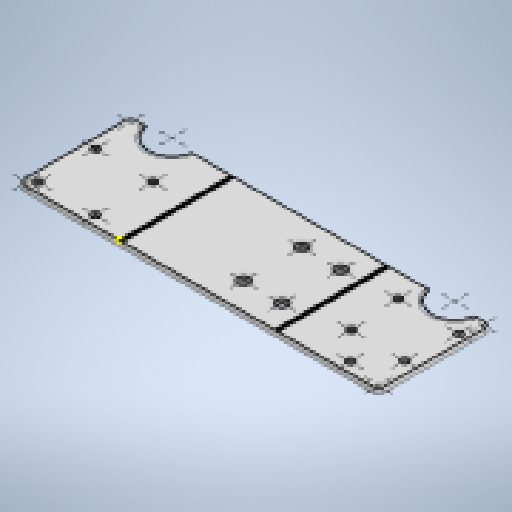
# Autodesk Inventor part: axis_22_bottom_frame
Saved by Autodesk Inventor 2026.1 (Build 301233000, 233)
## iProperties
Created: 2025-08-10
Part Number: axis_22_bottom_frame
Material: Generic
Document SubType Name: Modeling
Designer: LG
Density: 1 g/cm^3
Appearance: Default
Author: LG
Autodesk Inventor part; units mm, degrees
ref_plane "YZ Plane" through (0, 0, 0) normal (1, 0, 0) x (0, 1, 0)
ref_plane "XZ Plane" through (0, 0, 0) normal (0, 1, 0) x (-1, 0, 0)
ref_plane "XY Plane" through (0, 0, 0) normal (0, 0, 1) x (1, 0, 0)
sketch "Sketch1" plane through (0, 0, 0) normal (0, 1, 0) x (-1, 0, 0)
  line L0 (-0.4496, -29.3) -> (-0.4496, 0)
  line L1 (-41.2289, 0) -> (-41.2289, -29.3)
  circle A0 centre (-49.9386, -23.2) radius 1.05
  circle A1 centre (-50.9386, -9.98) radius 1.05
  circle A2 centre (-57.9386, -2.68) radius 1.05
  circle A3 centre (-64.9386, -9.98) radius 1.05
  circle A4 centre (-65.9386, -23.2) radius 1.05
  circle A5 centre (23.785, -2.5) radius 1.05
  circle A6 centre (8.735, -2.5) radius 1.05
  circle A7 centre (23.785, -17.6) radius 1.05
  circle A8 centre (8.735, -17.6) radius 1.05
  circle A9 centre (-25.6393, -7) radius 1.55
  circle A10 centre (-35.7793, -7) radius 1.55
  circle A11 centre (-25.6393, -22.3) radius 1.55
  circle A12 centre (-35.7793, -22.3) radius 1.55
  arc A13 (-67.0086, 0) -> (-68.0086, -1) centre (-67.0086, -1) ccw
  line L2 (-67.0086, 0) -> (25.33, 0)
  line L3 (-68.0086, -28.3) -> (-68.0086, -1)
  arc A14 (-68.0086, -28.3) -> (-67.0086, -29.3) centre (-67.0086, -28.3) ccw
  line L4 (-63.885, -29.3) -> (-67.0086, -29.3)
  arc A15 (-51.9921, -29.3) -> (-63.885, -29.3) centre (-57.9386, -30.1) ccw
  line L5 (10.3136, -29.3) -> (-51.9921, -29.3)
  arc A16 (22.2064, -29.3) -> (10.3136, -29.3) centre (16.26, -30.1) ccw
  line L6 (25.33, -29.3) -> (22.2064, -29.3)
  arc A17 (25.33, -29.3) -> (26.33, -28.3) centre (25.33, -28.3) ccw
  line L7 (26.33, -1) -> (26.33, -28.3)
  arc A18 (26.33, -1) -> (25.33, 0) centre (25.33, -1) ccw
  line L8 (-41.6786, -29.3) -> (-41.6786, 0)
  line L9 (-40.7793, 0) -> (-40.7793, -29.3)
  line L10 (-0.8993, -29.3) -> (-0.8993, 0)
  line L11 (0, 0) -> (0, -29.3)
  point P0 (0, 0)
  constraints: 24 end point, 19 centre point, 15 equal radius, 12 point on circle, 12 point on line, 11 tangent, 8 vertical, 7 parallel, 4 horizontal, 2 perpendicular, 1 collinear, 63 other
extrude "Extrusion1" add sketch "Sketch1" against normal blind 1.5
sketch "Sketch2" plane through (0, 0, 0) normal (0, 1, 0) x (1, 0, 0)
  circle A0 centre (-16.26, 30.1) radius 6.75
  circle A1 centre (57.9386, 30.1) radius 6.75
  point P0 (0, 0)
  dimension "d2" = 13.5
  dimension "d3" = 13.5
  constraints: 2 centre point, 2 coincident
  measures "d2" diameter of A0
  measures "d3" diameter of A1
extrude "Extrusion2" cut sketch "Sketch2" against normal blind 10
body "Solid1"
